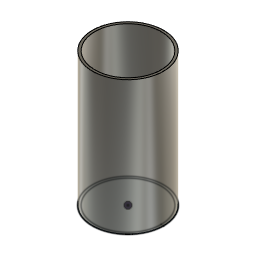
Top and Bottom Can Design Base (Autodesk Fusion 360 design; units mm, degrees)
Autodesk Fusion 360 part; units mm, degrees
sketch "Base" plane through (0, 0, 0) normal (0, 0, 1) x (1, 0, 0)
  circle A0 centre (0, 0) radius 30
  circle A1 centre (0, 0) radius 28
  dimension "d1" = 60
  dimension "d2" = 56
  constraint coincident A0.centre A1.centre
  constraint concentric A0 A1
  measures "d1" diameter of A0
  measures "d2" diameter of A1
extrude "Extrude1" add sketch "Base" along normal blind 2 contours A1
extrude "Extrude2" add sketch "Base" along normal blind 113
named bodies: "Bottom"
